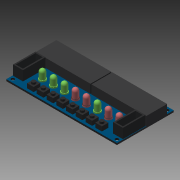
# Autodesk Inventor part: tm1638module
Saved by Autodesk Inventor 2014 (Build 180170000, 170)
## iProperties
Created: 2014-05-20
Part Number: tm1638module
Material: Generic
Document SubType Name: Modeling
Designer: brent
Density: 1 g/cm^3
Appearance: Default
Author: brent
Autodesk Inventor part; units mm, degrees
ref_plane "YZ Plane" through (0, 0, 0) normal (1, 0, 0) x (0, 1, 0)
ref_plane "XZ Plane" through (0, 0, 0) normal (0, 1, 0) x (-1, 0, 0)
ref_plane "XY Plane" through (0, 0, 0) normal (0, 0, 1) x (1, 0, 0)
sketch "Sketch1" plane through (0, 0, 0) normal (0, 1, 0) x (-1, 0, 0)
  line L0 (0, 0) -> (100.838, 0)
  line L1 (100.838, 0) -> (100.838, -51.7144)
  line L2 (100.838, -51.7144) -> (0, -51.7144)
  line L3 (0, -51.7144) -> (0, 0)
  dimension "d0" = 51.7144
  dimension "d1" = 100.838
  constraints: 8 end point, 2 parallel, 1 coincident, 1 horizontal, 1 perpendicular
  measures "d0" distance between parallel lines of L2 L0
  measures "d1" distance between parallel lines of L1 L3
extrude "Extrusion1" add sketch "Sketch1" along normal blind 1.524
sketch "Sketch2" plane through (0, 1.524, 0) normal (0, 1, 0) x (1, 0, 0)
  line L0 (-100.838, 0) -> (0, 0) projected
  line L1 (0, 0) -> (0, 51.7144) projected
  line L2 (0, 51.7144) -> (-100.838, 51.7144) projected
  line L3 (-100.838, 51.7144) -> (-100.838, 0) projected
  circle A0 centre (-97.838, 48.7144) radius 1.5
  circle A1 centre (-97.838, 3) radius 1.5
  circle A2 centre (-3, 3) radius 1.5
  circle A3 centre (-3, 48.7144) radius 1.5
  dimension "d4" = 3
  dimension "d5" = 3
  dimension "d6" = 3
  dimension "d7" = 3
  dimension "d8" = 3
  dimension "d9" = 3
  dimension "d10" = 3
  dimension "d11" = 3
  dimension "d12" = 3
  dimension "d13" = 3
  dimension "d14" = 3
  dimension "d15" = 3
  constraints: 4 centre point
  measures "d4" diameter of A0
  measures "d5" distance from line of L2 A0.centre
  measures "d6" distance from line of L3 A0.centre
  measures "d7" diameter of A1
  measures "d8" diameter of A2
  measures "d9" diameter of A3
  measures "d10" distance from line of L3 A1.centre
  measures "d11" distance from line of L0 A1.centre
  measures "d12" distance from line of L0 A2.centre
  measures "d13" distance from line of L1 A2.centre
  measures "d14" distance from line of L2 A3.centre
  measures "d15" distance from line of L1 A3.centre
extrude "Extrusion2" cut sketch "Sketch2" against normal through all contours A0 | A1 | A2 | A3
sketch "Sketch3" plane through (0, 1.524, 0) normal (0, 1, 0) x (1, 0, 0)
  line L0 (0, 0) -> (0, 51.7144) projected
  line L1 (0, 51.7144) -> (-100.838, 51.7144) projected
  line L2 (-100.838, 51.7144) -> (-100.838, 0) projected
  line L3 (-100.838, 45.7144) -> (-50.838, 45.7144)
  line L4 (-50.838, 45.7144) -> (-50.838, 26.7144)
  line L5 (-50.838, 26.7144) -> (-100.838, 26.7144)
  line L6 (-100.838, 26.7144) -> (-100.838, 45.7144)
  line L7 (0, 45.7144) -> (-50, 45.7144)
  line L8 (-50, 45.7144) -> (-50, 26.7144)
  line L9 (-50, 26.7144) -> (0, 26.7144)
  line L10 (0, 26.7144) -> (0, 45.7144)
  dimension "d18" = 6
  dimension "d19" = 6
  dimension "d20" = 19
  dimension "d21" = 50
  dimension "d22" = 50
  constraints: 16 end point, 4 parallel, 3 point on line, 2 horizontal, 2 perpendicular
  measures "d18" distance between parallel lines of L1 L3
  measures "d19" distance between parallel lines of L1 L7
  measures "d20" distance between parallel lines of L3 L5
  measures "d21" distance between parallel lines of L2 L4
  measures "d22" distance between parallel lines of L0 L8
extrude "Extrusion3" add sketch "Sketch3" along normal blind 8
sketch "Sketch4" plane through (0, 1.524, 0) normal (0, 1, 0) x (1, 0, 0)
  line L0 (-100.838, 26.7144) -> (-100.838, 0) projected
  line L1 (-100.838, 0) -> (0, 0) projected
  line L2 (-84.188, 8.3) -> (-78.188, 8.3)
  line L3 (-78.188, 8.3) -> (-78.188, 2.3)
  line L4 (-78.188, 2.3) -> (-84.188, 2.3)
  line L5 (-84.188, 2.3) -> (-84.188, 8.3)
  dimension "d25" = 6
  dimension "d26" = 6
  dimension "d27" = 2.3
  dimension "d28" = 16.65
  constraints: 8 end point, 2 parallel, 1 horizontal, 1 perpendicular
  measures "d25" distance of L3.end L4.end
  measures "d26" distance of L2.end L3.end
  measures "d27" distance between parallel lines of L1 L4
  measures "d28" distance between parallel lines of L0 L5
extrude "Extrusion4" add sketch "Sketch4" along normal blind 4
sketch "Sketch5" plane through (0, 5.524, 0) normal (0, 1, 0) x (1, 0, 0)
  circle A0 centre (-81.188, 5.3) radius 1.725
  point P0 (0, 0)
  dimension "d31" = 3.45
  constraints: 1 centre point
  measures "d31" diameter of A0
extrude "Extrusion5" add sketch "Sketch5" along normal blind 1.65
pattern_linear "Rectangular Pattern1" count 8 spacing 8.88 along (1, 0, 0) of "Extrusion4", "Extrusion5"
sketch "Sketch6" plane through (0, 1.524, 0) normal (0, 1, 0) x (1, 0, 0)
  line L0 (-100.838, 26.7144) -> (-100.838, 0) projected
  line L1 (-100.838, 0) -> (0, 0) projected
  circle A0 centre (-83.838, 16) radius 2.5
  dimension "d37" = 5
  dimension "d38" = 17
  dimension "d39" = 16
  constraints: 1 centre point
  measures "d37" diameter of A0
  measures "d38" distance from line of L0 A0.centre
  measures "d39" distance from line of L1 A0.centre
extrude "Extrusion6" add sketch "Sketch6" along normal blind 9
fillet "Fillet1" radius 2.5 1 edges at (-86.338, 10.524, -16)
sketch "Sketch7" plane through (0, 1.524, 0) normal (0, 1, 0) x (1, 0, 0)
  circle A0 centre (-83.838, 16) radius 2.5 projected
  line L0 (0, 0) -> (0, 26.7144) projected
  arc A1 (-86.338, 14.5303) -> (-86.338, 17.4697) centre (-83.838, 16) ccw
  line L1 (-86.338, 17.4697) -> (-86.338, 14.5303)
  circle A2 centre (-83.838, 16) radius 2.5 projected
  dimension "d43" = 5.8
  constraints: 2 end point, 2 point on circle, 1 centre point, 1 coincident, 1 parallel, 1 tangent
  measures "d43" diameter of A1
extrude "Extrusion7" add sketch "Sketch7" along normal blind 1.2 contours A0 | L1 A1
pattern_linear "Rectangular Pattern2" count 8 spacing 10 along (1, 0, 0) of "Extrusion7", "Extrusion6", "Fillet1"
sketch "Sketch8" plane through (0, 1.524, 0) normal (0, 1, 0) x (1, 0, 0)
  line L0 (-50.838, 26.7144) -> (-100.838, 26.7144) projected
  line L1 (-100.838, 26.7144) -> (-100.838, 0) projected
  line L2 (0, 0) -> (0, 26.7144) projected
  line L3 (-100.438, 26.3144) -> (-91.438, 26.3144)
  line L4 (-91.438, 26.3144) -> (-91.438, 5.8144)
  line L5 (-91.438, 5.8144) -> (-100.438, 5.8144)
  line L6 (-100.438, 5.8144) -> (-100.438, 26.3144)
  line L7 (-99.168, 25.0444) -> (-92.708, 25.0444)
  line L8 (-92.708, 25.0444) -> (-92.708, 7.0844)
  line L9 (-92.708, 7.0844) -> (-99.168, 7.0844)
  line L10 (-99.168, 7.0844) -> (-99.168, 25.0444)
  line L11 (-0.4, 26.3144) -> (-9.4, 26.3144)
  line L12 (-9.4, 26.3144) -> (-9.4, 5.8144)
  line L13 (-9.4, 5.8144) -> (-0.4, 5.8144)
  line L14 (-0.4, 5.8144) -> (-0.4, 26.3144)
  line L15 (-1.67, 25.0444) -> (-8.13, 25.0444)
  line L16 (-8.13, 25.0444) -> (-8.13, 7.0844)
  line L17 (-8.13, 7.0844) -> (-1.67, 7.0844)
  line L18 (-1.67, 7.0844) -> (-1.67, 25.0444)
  dimension "d49" = 9
  dimension "d50" = 0.4
  dimension "d51" = 0.4
  dimension "d52" = 20.5
  dimension "d53" = 1.27
  dimension "d54" = 1.27
  dimension "d55" = 1.27
  dimension "d56" = 1.27
  dimension "d57" = 1.27
  dimension "d58" = 0.4
  dimension "d59" = 9
  dimension "d60" = 1.27
  constraints: 32 end point, 8 parallel, 4 horizontal, 4 perpendicular, 4 point on line
  measures "d49" distance between parallel lines of L4 L6
  measures "d50" distance between parallel lines of L0 L3
  measures "d51" distance between parallel lines of L1 L6
  measures "d52" distance between parallel lines of L5 L3
  measures "d53" distance between parallel lines of L4 L8
  measures "d54" distance between parallel lines of L3 L7
  measures "d55" distance between parallel lines of L6 L10
  measures "d56" distance between parallel lines of L5 L9
  measures "d57" distance between parallel lines of L14 L18
  measures "d58" distance between parallel lines of L2 L14
  measures "d59" distance between parallel lines of L14 L12
  measures "d60" distance between parallel lines of L12 L16
extrude "Extrusion8" add sketch "Sketch8" along normal blind 8.86
body "Solid1"
